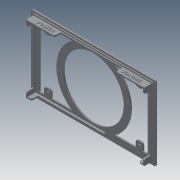
# Autodesk Inventor part: upper
Saved by Autodesk Inventor 2014 (Build 180170000, 170)
## iProperties
Created: 2014-09-06
Part Number: upper
Material: 一般
Document SubType Name: Modeling
Designer: Hideyuki Takei
Density: 1 g/cm^3
Appearance: 既定
Author: Hideyuki Takei
Autodesk Inventor part; units mm, degrees
ref_plane "YZ Plane" through (0, 0, 0) normal (1, 0, 0) x (0, 1, 0)
ref_plane "XZ Plane" through (0, 0, 0) normal (0, 1, 0) x (-1, 0, 0)
ref_plane "XY Plane" through (0, 0, 0) normal (0, 0, 1) x (1, 0, 0)
sketch "スケッチ2" plane through (0, 0, 0) normal (0, 1, 0) x (-1, 0, 0)
  line L0 (0, 0) -> (136, 0)
  line L1 (136, 0) -> (136, 81)
  line L2 (136, 81) -> (0, 81)
  line L3 (0, 81) -> (0, 0)
  dimension "d2" = 81
  dimension "d3" = 136
  constraints: 8 end point, 2 parallel, 1 horizontal, 1 perpendicular
  measures "d2" distance of L2.end L0.start
  measures "d3" distance of L1.end L2.end
extrude "押し出し1" add sketch "スケッチ2" along normal blind 1.5
sketch "スケッチ3" plane through (0, 0, 0) normal (0, 1, 0) x (-1, 0, 0)
  line L0 (5, 5) -> (131, 5)
  line L1 (131, 5) -> (131, 76)
  line L2 (131, 76) -> (5, 76)
  line L3 (5, 76) -> (5, 5)
  line L4 (136, 0) -> (136, 81) projected
  line L5 (136, 81) -> (0, 81) projected
  line L6 (132.5, 77.5) -> (126.5, 77.5)
  line L7 (126.5, 77.5) -> (126.5, 76)
  line L8 (126.5, 76) -> (132.5, 76)
  line L9 (132.5, 76) -> (132.5, 77.5)
  line L10 (131, 76) -> (132.5, 76)
  line L11 (132.5, 76) -> (132.5, 71)
  line L12 (132.5, 71) -> (131, 71)
  line L13 (131, 71) -> (131, 76)
  line L14 (131, 5) -> (132.5, 5)
  line L15 (132.5, 5) -> (132.5, 10)
  line L16 (132.5, 10) -> (131, 10)
  line L17 (131, 10) -> (131, 5)
  line L18 (132.5, 5) -> (126.5, 5)
  line L19 (126.5, 5) -> (126.5, 3.5)
  line L20 (126.5, 3.5) -> (132.5, 3.5)
  line L21 (132.5, 3.5) -> (132.5, 5)
  line L22 (5, 76) -> (3.5, 76)
  line L23 (3.5, 76) -> (3.5, 71)
  line L24 (3.5, 71) -> (5, 71)
  line L25 (5, 71) -> (5, 76)
  line L26 (3.5, 76) -> (9.5, 76)
  line L27 (9.5, 76) -> (9.5, 77.5)
  line L28 (9.5, 77.5) -> (3.5, 77.5)
  line L29 (3.5, 77.5) -> (3.5, 76)
  line L30 (5, 5) -> (3.5, 5)
  line L31 (3.5, 5) -> (3.5, 10)
  line L32 (3.5, 10) -> (5, 10)
  line L33 (5, 10) -> (5, 5)
  line L34 (3.5, 5) -> (9.5, 5)
  line L35 (9.5, 5) -> (9.5, 3.5)
  line L36 (9.5, 3.5) -> (3.5, 3.5)
  line L37 (3.5, 3.5) -> (3.5, 5)
  point P0 (0, 0)
  dimension "d6" = 126
  dimension "d7" = 71
  dimension "d8" = 5
  dimension "d9" = 5
  dimension "d10" = 1.5
  dimension "d11" = 1.5
  dimension "d12" = 5
  dimension "d13" = 6
  dimension "d14" = 0
  dimension "d17" = 1.5
  dimension "d18" = 1.5
  dimension "d19" = 6
  dimension "d20" = 5
  dimension "d21" = 5
  dimension "d22" = 1.5
  dimension "d23" = 1.5
  dimension "d24" = 6
  dimension "d25" = 6
  dimension "d26" = 1.5
  dimension "d27" = 1.5
  dimension "d28" = 5
  constraints: 72 end point, 18 parallel, 9 horizontal, 9 perpendicular, 1 point on line
  measures "d6" distance of L1.end L2.end
  measures "d7" distance of L0.end L1.end
  measures "d8" distance between parallel lines of L4 L1
  measures "d9" distance between parallel lines of L5 L2
  measures "d10" distance of L11.end L12.end
  measures "d11" distance of L8.end L6.start
  measures "d12" distance of L10.end L11.end
  measures "d13" distance of L6.start L6.end
  measures "d14" distance between parallel lines of L11 L9
  measures "d17" distance of L15.end L16.end
  measures "d18" distance of L20.end L14.end
  measures "d19" distance of L19.end L20.end
  measures "d20" distance of L14.end L15.end
  measures "d21" distance of L22.end L23.end
  measures "d22" distance of L23.end L24.end
  measures "d23" distance of L28.end L22.end
  measures "d24" distance of L27.end L28.end
  measures "d25" distance of L35.end L36.end
  measures "d26" distance of L34.end L35.end
  measures "d27" distance of L31.end L32.end
  measures "d28" distance of L30.end L31.end
extrude "押し出し2" add sketch "スケッチ3" against normal blind 9.01 contours L30 L31 L32 L3 | L0 L35 L36 L37 L30 | L0 L14 L21 L20 L19 | L24 L23 L22 L3 | L1 L16 L15 L14 | L22 L29 L28 L27 L2 | L1 L8 L11 L12 | L7 L6 L9 L8 L2
sketch "スケッチ5" plane through (0, 0, 0) normal (0, 1, 0) x (-1, 0, 0)
  line L0 (131, 76) -> (5, 76)
  line L1 (5, 76) -> (5, 5)
  line L2 (5, 5) -> (131, 5)
  line L3 (131, 5) -> (131, 76)
  line L4 (0, 81) -> (0, 0) projected
  line L5 (131, 76) -> (5, 76)
  line L6 (5, 76) -> (5, 77.5)
  line L7 (5, 77.5) -> (131, 77.5)
  line L8 (131, 77.5) -> (131, 76)
  line L9 (131, 5) -> (5, 5)
  line L10 (5, 5) -> (5, 3.5)
  line L11 (5, 3.5) -> (131, 3.5)
  line L12 (131, 3.5) -> (131, 5)
  line L13 (131, 77.5) -> (132.5, 77.5)
  line L14 (132.5, 77.5) -> (132.5, 3.5)
  line L15 (132.5, 3.5) -> (131, 3.5)
  line L16 (131, 3.5) -> (131, 77.5)
  line L17 (5, 77.5) -> (3.5, 77.5)
  line L18 (3.5, 77.5) -> (3.5, 3.5)
  line L19 (3.5, 3.5) -> (5, 3.5)
  line L20 (5, 3.5) -> (5, 77.5)
  dimension "d34" = 126
  dimension "d35" = 71
  dimension "d36" = 5
  dimension "d37" = 5
  dimension "d38" = 1.5
  dimension "d39" = 1.5
  dimension "d40" = 1.5
  dimension "d41" = 1.5
  dimension "d42" = 1.5
  dimension "d43" = 1.5
  constraints: 40 end point, 10 parallel, 5 horizontal, 5 perpendicular
  measures "d34" distance of L0.start L0.end
  measures "d35" distance of L2.end L0.start
  measures "d36" distance from line of L4.end L2
  measures "d37" distance between parallel lines of L4 L1
  measures "d38" distance of L5.end L6.end
  measures "d39" distance of L9.end L10.end
  measures "d40" distance of L14.end L15.end
  measures "d41" distance of L18.end L19.end
  measures "d42" distance between parallel lines of L19 L2
  measures "d43" distance between parallel lines of L18 L1
extrude "押し出し4" add sketch "スケッチ5" against normal blind 2 contours L8 L13 L14 L15 L12 L3 | L0 L6 L7 L8 | L1 L10 L19 L18 L17 L6 | L12 L11 L10 L2
sketch "スケッチ6" plane through (0, -2, 0) normal (0, -1, 0) x (1, 0, 0)
  line L0 (-126.5, 76) -> (-126.5, 77.5) projected
  line L1 (-126.5, 76) -> (-9.5, 76) projected
  line L2 (-9.5, 77.5) -> (-126.5, 77.5) projected
  line L3 (-126.5, 77.5) -> (-101.5, 77.5)
  line L4 (-101.5, 77.5) -> (-101.5, 76)
  line L5 (-101.5, 76) -> (-126.5, 76)
  line L6 (-126.5, 76) -> (-126.5, 77.5)
  line L7 (-9.5, 76) -> (-34.5, 76)
  line L8 (-34.5, 76) -> (-34.5, 77.5)
  line L9 (-34.5, 77.5) -> (-9.5, 77.5)
  line L10 (-9.5, 77.5) -> (-9.5, 76)
  point P0 (0, 0)
  dimension "d46" = 25
  dimension "d47" = 25
  constraints: 16 end point, 4 parallel, 2 horizontal, 2 perpendicular, 2 point on line
  measures "d46" distance of L0.end L3.end
  measures "d47" distance of L8.end L9.end
extrude "押し出し5" add sketch "スケッチ6" along normal blind 7 contours L0 L2 L4 L1 | L8 L2 L10 L1
sketch "スケッチ7" plane through (0, 0, 0) normal (0, 1, 0) x (-1, 0, 0)
  line L0 (9, 73.5) -> (127, 73.5)
  line L1 (127, 73.5) -> (127, 7.5)
  line L2 (127, 7.5) -> (9, 7.5)
  line L3 (9, 7.5) -> (9, 73.5)
  line L4 (136, 0) -> (136, 81) projected
  line L5 (136, 81) -> (0, 81) projected
  point P0 (0, 0)
  dimension "d50" = 66
  dimension "d51" = 118
  dimension "d52" = 9
  dimension "d53" = 7.5
  constraints: 8 end point, 2 parallel, 1 horizontal, 1 perpendicular
  measures "d50" distance of L0.end L1.end
  measures "d51" distance of L1.end L2.end
  measures "d52" distance between parallel lines of L1 L4
  measures "d53" distance between parallel lines of L5 L0
extrude "押し出し6" cut sketch "スケッチ7" along normal up to next
sketch "スケッチ8" plane through (0, 0, 0) normal (0, 1, 0) x (-1, 0, 0)
  circle A0 centre (68, 40.5) radius 33
  circle A1 centre (68, 40.5) radius 40.5
  line L0 (0, 81) -> (0, 0) projected
  line L1 (0, 0) -> (136, 0) projected
  dimension "d56" = 66
  dimension "d57" = 81
  dimension "d58" = 68
  dimension "d59" = 40.5
  constraints: 2 centre point, 1 coincident
  measures "d56" diameter of A0
  measures "d57" diameter of A1
  measures "d58" distance from line of L0 A0.centre
  measures "d59" distance from line of L1 A0.centre
extrude "押し出し7" add sketch "スケッチ8" along normal blind 1.5
sketch "スケッチ9" plane through (-132.5, 0, 77.5) normal (0, 0, 1) x (1, 0, 0)
  line L0 (129, 0) -> (129, -9.01) projected
  line L1 (0, 0) -> (129, 0) projected
  line L2 (0, 0) -> (129, 0)
  line L3 (129, 0) -> (129, -1)
  line L4 (129, -1) -> (0, -1)
  line L5 (0, -1) -> (0, 0)
  point P0 (132.5, 0)
  dimension "d62" = 1
  constraints: 8 end point, 2 parallel, 1 horizontal, 1 perpendicular, 1 point on line
  measures "d62" distance of L4.end L1.start
extrude "押し出し8" add sketch "スケッチ9" along normal blind 1.5
sketch "スケッチ10" plane through (-3.5, 0, 3.5) normal (0, 0, -1) x (-1, 0, 0)
  line L0 (129, 0) -> (129, -9.01) projected
  line L1 (0, 0) -> (129, 0)
  line L2 (129, 0) -> (129, -1)
  line L3 (129, -1) -> (0, -1)
  line L4 (0, -1) -> (0, 0)
  point P0 (-3.5, 0)
  dimension "d65" = 1
  constraints: 8 end point, 2 parallel, 1 horizontal, 1 perpendicular, 1 point on line
  measures "d65" distance of L1.end L2.end
extrude "押し出し9" add sketch "スケッチ10" along normal blind 1.5
sketch "スケッチ11" plane through (-3.5, -9.01, 10) normal (1, 0, 0) x (0, 0, -1)
  line L0 (-69, 9.01) -> (8, 9.01)
  line L1 (8, 9.01) -> (8, 8.01)
  line L2 (8, 8.01) -> (-69, 8.01)
  line L3 (-69, 8.01) -> (-69, 9.01)
  point P0 (10, 9.01)
  constraints: 8 end point, 2 parallel, 1 horizontal, 1 perpendicular
extrude "押し出し10" add sketch "スケッチ11" along normal blind 1.5
sketch "スケッチ12" plane through (-132.5, -9.01, 3.5) normal (-1, 0, 0) x (0, 0, 1)
  line L0 (-1.5, 9.01) -> (75.5, 9.01)
  line L1 (75.5, 9.01) -> (75.5, 8.01)
  line L2 (75.5, 8.01) -> (-1.5, 8.01)
  line L3 (-1.5, 8.01) -> (-1.5, 9.01)
  point P0 (-3.5, 9.01)
  constraints: 8 end point, 2 parallel, 1 horizontal, 1 perpendicular
extrude "押し出し11" add sketch "スケッチ12" along normal blind 1.5
sketch "スケッチ13" plane through (0, 1.5, 0) normal (0, 1, 0) x (1, 0, 0)
  line L0 (-44.5213, -7.5) -> (-9, -7.5) projected
  line L1 (-9, -7.5) -> (-9, -73.5) projected
  line L2 (-9, -73.5) -> (-44.5213, -73.5) projected
  line L3 (-91.4787, -73.5) -> (-127, -73.5) projected
  line L4 (-127, -73.5) -> (-127, -7.5) projected
  line L5 (-127, -7.5) -> (-91.4787, -7.5) projected
  line L6 (-122, -7.5) -> (-114, -7.5)
  line L7 (-114, -7.5) -> (-114, -15.5)
  line L8 (-114, -15.5) -> (-122, -15.5)
  line L9 (-122, -15.5) -> (-122, -7.5)
  line L10 (-122, -73.5) -> (-114, -73.5)
  line L11 (-114, -73.5) -> (-114, -65.5)
  line L12 (-114, -65.5) -> (-122, -65.5)
  line L13 (-122, -65.5) -> (-122, -73.5)
  line L14 (-14, -7.5) -> (-22, -7.5)
  line L15 (-22, -7.5) -> (-22, -15.5)
  line L16 (-22, -15.5) -> (-14, -15.5)
  line L17 (-14, -15.5) -> (-14, -7.5)
  line L18 (-14, -73.5) -> (-22, -73.5)
  line L19 (-22, -73.5) -> (-22, -65.5)
  line L20 (-22, -65.5) -> (-14, -65.5)
  line L21 (-14, -65.5) -> (-14, -73.5)
  circle A0 centre (-118, -12.5) radius 1.25
  circle A1 centre (-118, -68.5) radius 1.25
  circle A2 centre (-18, -12.5) radius 1.25
  circle A3 centre (-18, -68.5) radius 1.25
  dimension "d72" = 8
  dimension "d73" = 8
  dimension "d74" = 8
  dimension "d75" = 8
  dimension "d76" = 8
  dimension "d77" = 8
  dimension "d78" = 8
  dimension "d79" = 8
  dimension "d80" = 5
  dimension "d81" = 5
  dimension "d82" = 5
  dimension "d83" = 5
  dimension "d84" = 2.5
  dimension "d85" = 2.5
  dimension "d86" = 2.5
  dimension "d87" = 2.5
  dimension "d88" = 4
  dimension "d89" = 3
  dimension "d90" = 3
  dimension "d91" = 4
  dimension "d92" = 4
  dimension "d93" = 5
  dimension "d94" = 4
  dimension "d95" = 5
  constraints: 32 end point, 8 parallel, 4 centre point, 4 horizontal, 4 perpendicular, 4 point on line
  measures "d72" distance of L8.end L6.start
  measures "d73" distance of L12.end L10.start
  measures "d74" distance of L20.end L18.start
  measures "d75" distance of L16.end L14.start
  measures "d76" distance of L7.end L8.end
  measures "d77" distance of L11.end L12.end
  measures "d78" distance of L19.end L20.end
  measures "d79" distance of L15.end L16.end
  measures "d80" distance between parallel lines of L9 L4
  measures "d81" distance between parallel lines of L4 L13
  measures "d82" distance between parallel lines of L1 L17
  measures "d83" distance between parallel lines of L1 L21
  measures "d84" diameter of A3
  measures "d85" diameter of A1
  measures "d86" diameter of A0
  measures "d87" diameter of A2
  measures "d88" distance from line of L9 A0.centre
  measures "d89" distance from line of L8 A0.centre
  measures "d90" distance from line of L16 A2.centre
  measures "d91" distance from line of L15 A2.centre
  measures "d92" distance from line of L19 A3.centre
  measures "d93" distance from line of L2 A3.centre
  measures "d94" distance from line of L13 A1.centre
  measures "d95" distance from line of L3 A1.centre
extrude "押し出し12" add sketch "スケッチ13" against normal blind 1.5
fillet "フィレット1" radius 3 8 edges at (-14, 0.75, 65.5) (-22, 0.75, 65.5) (-114, 0.75, 65.5) (-122, 0.75, 65.5) (-114, 0.75, 15.5) (-122, 0.75, 15.5) (-14, 0.75, 15.5) (-22, 0.75, 15.5)
fillet "フィレット2" radius 1.5 8 edges at (0, 0.75, 81) (0, 0.75, 0) (-136, 0.75, 0) (-136, 0.75, 81) (-134, -0.5, 79) (-134, -0.5, 2) (-2, -0.5, 2) (-2, -0.5, 79)
sketch "スケッチ14" plane through (-9.5, -9.01, 77.5) normal (0, 0, 1) x (1, 0, 0)
  line L0 (6, 8.01) -> (-123, 8.01) projected
  line L1 (-123, 8.01) -> (-123, 0) projected
  line L2 (-114, 5.51) -> (-95.7285, 5.51) construction
  line L3 (-95.7285, 5.51) -> (-95.7285, 1.8625) construction
  line L4 (-95.7285, 1.8625) -> (-114, 1.8625) construction
  line L5 (-114, 1.8625) -> (-114, 5.51) construction
  line L6 (6, 8.01) -> (6, 0) projected
  line L7 (-22, 5.51) -> (-1.4737, 5.51) construction
  line L8 (-1.4737, 5.51) -> (-1.4737, 32.8525) construction
  line L9 (-1.4737, 32.8525) -> (-22, 32.8525) construction
  line L10 (-22, 32.8525) -> (-22, 5.51) construction
  spline S0 degree 2 poles (-110.9453, 4.3329) (-110.9453, 4.089) (-111.1013, 3.6465) (-111.2459, 3.4991) knots 0 0 0 1 2 2 2
  spline S1 degree 2 poles (-111.2459, 3.4991) (-111.3339, 3.4055) (-111.5494, 3.2523) (-111.6771, 3.1984) knots 0 0 0 1 2 2 2
  spline S2 degree 2 poles (-111.6771, 3.1984) (-111.8075, 3.1445) (-112.111, 3.0821) (-112.2982, 3.0821) knots 0 0 0 1 2 2 2
  line L11 (-112.2982, 3.0821) -> (-112.7577, 3.0821)
  line L12 (-112.7577, 3.0821) -> (-112.7577, 1.9363)
  line L13 (-112.7577, 1.9363) -> (-113.637, 1.9363)
  line L14 (-113.637, 1.9363) -> (-113.637, 5.4363)
  line L15 (-113.637, 5.4363) -> (-112.2784, 5.4363)
  spline S3 degree 2 poles (-112.2784, 5.4363) (-111.9777, 5.4363) (-111.5381, 5.3256) (-111.3594, 5.2065) knots 0 0 0 1 2 2 2
  spline S4 degree 2 poles (-111.3594, 5.2065) (-111.1609, 5.0732) (-110.9453, 4.6364) (-110.9453, 4.3329) knots 0 0 0 1 2 2 2
  spline S5 degree 2 poles (-111.8472, 4.3102) (-111.8472, 4.4606) (-111.9891, 4.6733) (-112.0855, 4.713) knots 0 0 0 1 2 2 2
  spline S6 degree 2 poles (-112.0855, 4.713) (-112.2103, 4.7669) (-112.4372, 4.7839) (-112.6329, 4.7839) knots 0 0 0 1 2 2 2
  line L16 (-112.6329, 4.7839) -> (-112.7577, 4.7839)
  line L17 (-112.7577, 4.7839) -> (-112.7577, 3.7345)
  line L18 (-112.7577, 3.7345) -> (-112.6953, 3.7345)
  spline S7 degree 2 poles (-112.6953, 3.7345) (-112.5733, 3.7345) (-112.3521, 3.7401) (-112.2699, 3.7543) knots 0 0 0 1 2 2 2
  spline S8 degree 2 poles (-112.2699, 3.7543) (-112.1989, 3.7657) (-112.0429, 3.8337) (-112.0004, 3.8763) knots 0 0 0 1 2 2 2
  spline S9 degree 2 poles (-112.0004, 3.8763) (-111.9096, 3.9614) (-111.8472, 4.1514) (-111.8472, 4.3102) knots 0 0 0 1 2 2 2
  spline S10 degree 2 poles (-107.2893, 3.6863) (-107.2893, 2.8354) (-108.1969, 1.8625) (-108.9854, 1.8625) knots 0 0 0 1 2 2 2
  spline S11 degree 2 poles (-108.9854, 1.8625) (-109.7767, 1.8625) (-110.6787, 2.8467) (-110.6787, 3.6863) knots 0 0 0 1 2 2 2
  spline S12 degree 2 poles (-110.6787, 3.6863) (-110.6787, 4.5286) (-109.7767, 5.51) (-108.9854, 5.51) knots 0 0 0 1 2 2 2
  spline S13 degree 2 poles (-108.9854, 5.51) (-108.1969, 5.51) (-107.2893, 4.5343) (-107.2893, 3.6863) knots 0 0 0 1 2 2 2
  spline S14 degree 2 poles (-108.1969, 3.6863) (-108.1969, 4.0011) (-108.3246, 4.4407) (-108.4352, 4.5797) knots 0 0 0 1 2 2 2
  spline S15 degree 2 poles (-108.4352, 4.5797) (-108.5458, 4.7243) (-108.8294, 4.8491) (-108.9826, 4.8491) knots 0 0 0 1 2 2 2
  spline S16 degree 2 poles (-108.9826, 4.8491) (-109.1442, 4.8491) (-109.408, 4.7329) (-109.53, 4.5854) knots 0 0 0 1 2 2 2
  spline S17 degree 2 poles (-109.53, 4.5854) (-109.6378, 4.4492) (-109.7711, 3.9982) (-109.7711, 3.6863) knots 0 0 0 1 2 2 2
  spline S18 degree 2 poles (-109.7711, 3.6863) (-109.7711, 3.3629) (-109.6434, 2.9375) (-109.5328, 2.7928) knots 0 0 0 1 2 2 2
  spline S19 degree 2 poles (-109.5328, 2.7928) (-109.4222, 2.6482) (-109.1357, 2.5234) (-108.9826, 2.5234) knots 0 0 0 1 2 2 2
  spline S20 degree 2 poles (-108.9826, 2.5234) (-108.8266, 2.5234) (-108.5373, 2.6567) (-108.4323, 2.7985) knots 0 0 0 1 2 2 2
  spline S21 degree 2 poles (-108.4323, 2.7985) (-108.3189, 2.9517) (-108.1969, 3.3572) (-108.1969, 3.6863) knots 0 0 0 1 2 2 2
  line L19 (-102.2549, 5.4363) -> (-103.1398, 1.9363)
  line L20 (-103.1398, 1.9363) -> (-104.1041, 1.9363)
  line L21 (-104.1041, 1.9363) -> (-104.6657, 4.1004)
  line L22 (-104.6657, 4.1004) -> (-105.2075, 1.9363)
  line L23 (-105.2075, 1.9363) -> (-106.1746, 1.9363)
  line L24 (-106.1746, 1.9363) -> (-107.0596, 5.4363)
  line L25 (-107.0596, 5.4363) -> (-106.1463, 5.4363)
  line L26 (-106.1463, 5.4363) -> (-105.6641, 3.0935)
  line L27 (-105.6641, 3.0935) -> (-105.0798, 5.4363)
  line L28 (-105.0798, 5.4363) -> (-104.2062, 5.4363)
  line L29 (-104.2062, 5.4363) -> (-103.6503, 3.0906)
  line L30 (-103.6503, 3.0906) -> (-103.1455, 5.4363)
  line L31 (-103.1455, 5.4363) -> (-102.2549, 5.4363)
  line L32 (-101.8209, 1.9363) -> (-101.8209, 5.4363)
  line L33 (-101.8209, 5.4363) -> (-99.4554, 5.4363)
  line L34 (-99.4554, 5.4363) -> (-99.4554, 4.7697)
  line L35 (-99.4554, 4.7697) -> (-100.9473, 4.7697)
  line L36 (-100.9473, 4.7697) -> (-100.9473, 4.1542)
  line L37 (-100.9473, 4.1542) -> (-99.5717, 4.1542)
  line L38 (-99.5717, 4.1542) -> (-99.5717, 3.4877)
  line L39 (-99.5717, 3.4877) -> (-100.9473, 3.4877)
  line L40 (-100.9473, 3.4877) -> (-100.9473, 2.6028)
  line L41 (-100.9473, 2.6028) -> (-99.4554, 2.6028)
  line L42 (-99.4554, 2.6028) -> (-99.4554, 1.9363)
  line L43 (-99.4554, 1.9363) -> (-101.8209, 1.9363)
  line L44 (-95.6264, 1.9363) -> (-96.6957, 1.9363)
  line L45 (-96.6957, 1.9363) -> (-97.6686, 3.2211)
  line L46 (-97.6686, 3.2211) -> (-97.9862, 3.2211)
  line L47 (-97.9862, 3.2211) -> (-97.9862, 1.9363)
  line L48 (-97.9862, 1.9363) -> (-98.8598, 1.9363)
  line L49 (-98.8598, 1.9363) -> (-98.8598, 5.4363)
  line L50 (-98.8598, 5.4363) -> (-97.453, 5.4363)
  spline S22 degree 2 poles (-97.453, 5.4363) (-97.1609, 5.4363) (-96.7297, 5.3625) (-96.5454, 5.2491) knots 0 0 0 1 2 2 2
  spline S23 degree 2 poles (-96.5454, 5.2491) (-96.3582, 5.1299) (-96.137, 4.7584) (-96.137, 4.4747) knots 0 0 0 1 2 2 2
  spline S24 degree 2 poles (-96.137, 4.4747) (-96.137, 4.0748) (-96.5, 3.5728) (-96.8035, 3.4253) knots 0 0 0 1 2 2 2
  line L51 (-96.8035, 3.4253) -> (-95.6264, 1.9363)
  spline S25 degree 2 poles (-97.0389, 4.3641) (-97.0389, 4.4974) (-97.141, 4.6875) (-97.2573, 4.7385) knots 0 0 0 1 2 2 2
  spline S26 degree 2 poles (-97.2573, 4.7385) (-97.3395, 4.7726) (-97.5409, 4.7924) (-97.6912, 4.7924) knots 0 0 0 1 2 2 2
  line L52 (-97.6912, 4.7924) -> (-97.9862, 4.7924)
  line L53 (-97.9862, 4.7924) -> (-97.9862, 3.8508)
  line L54 (-97.9862, 3.8508) -> (-97.7338, 3.8508)
  spline S27 degree 2 poles (-97.7338, 3.8508) (-97.5523, 3.8508) (-97.2942, 3.8961) (-97.2062, 3.9671) knots 0 0 0 1 2 2 2
  spline S28 degree 2 poles (-97.2062, 3.9671) (-97.1212, 4.0351) (-97.0389, 4.2166) (-97.0389, 4.3641) knots 0 0 0 1 2 2 2
  line L55 (-18.7156, 5.4363) -> (-19.9182, 1.9363)
  line L56 (-19.9182, 1.9363) -> (-20.8343, 1.9363)
  line L57 (-20.8343, 1.9363) -> (-22.0369, 5.4363)
  line L58 (-22.0369, 5.4363) -> (-21.1264, 5.4363)
  line L59 (-21.1264, 5.4363) -> (-20.3635, 3.0623)
  line L60 (-20.3635, 3.0623) -> (-19.6033, 5.4363)
  line L61 (-19.6033, 5.4363) -> (-18.7156, 5.4363)
  spline S29 degree 2 poles (-15.2042, 3.6863) (-15.2042, 2.8354) (-16.1118, 1.8625) (-16.9003, 1.8625) knots 0 0 0 1 2 2 2
  spline S30 degree 2 poles (-16.9003, 1.8625) (-17.6917, 1.8625) (-18.5936, 2.8467) (-18.5936, 3.6863) knots 0 0 0 1 2 2 2
  spline S31 degree 2 poles (-18.5936, 3.6863) (-18.5936, 4.5286) (-17.6917, 5.51) (-16.9003, 5.51) knots 0 0 0 1 2 2 2
  spline S32 degree 2 poles (-16.9003, 5.51) (-16.1118, 5.51) (-15.2042, 4.5343) (-15.2042, 3.6863) knots 0 0 0 1 2 2 2
  spline S33 degree 2 poles (-16.1118, 3.6863) (-16.1118, 4.0011) (-16.2395, 4.4407) (-16.3501, 4.5797) knots 0 0 0 1 2 2 2
  spline S34 degree 2 poles (-16.3501, 4.5797) (-16.4607, 4.7243) (-16.7443, 4.8491) (-16.8975, 4.8491) knots 0 0 0 1 2 2 2
  spline S35 degree 2 poles (-16.8975, 4.8491) (-17.0592, 4.8491) (-17.3229, 4.7329) (-17.4449, 4.5854) knots 0 0 0 1 2 2 2
  spline S36 degree 2 poles (-17.4449, 4.5854) (-17.5527, 4.4492) (-17.686, 3.9982) (-17.686, 3.6863) knots 0 0 0 1 2 2 2
  spline S37 degree 2 poles (-17.686, 3.6863) (-17.686, 3.3629) (-17.5583, 2.9375) (-17.4477, 2.7928) knots 0 0 0 1 2 2 2
  spline S38 degree 2 poles (-17.4477, 2.7928) (-17.3371, 2.6482) (-17.0506, 2.5234) (-16.8975, 2.5234) knots 0 0 0 1 2 2 2
  spline S39 degree 2 poles (-16.8975, 2.5234) (-16.7415, 2.5234) (-16.4522, 2.6567) (-16.3472, 2.7985) knots 0 0 0 1 2 2 2
  spline S40 degree 2 poles (-16.3472, 2.7985) (-16.2338, 2.9517) (-16.1118, 3.3572) (-16.1118, 3.6863) knots 0 0 0 1 2 2 2
  line L62 (-12.3481, 1.9363) -> (-14.6823, 1.9363)
  line L63 (-14.6823, 1.9363) -> (-14.6823, 5.4363)
  line L64 (-14.6823, 5.4363) -> (-13.8031, 5.4363)
  line L65 (-13.8031, 5.4363) -> (-13.8031, 2.6028)
  line L66 (-13.8031, 2.6028) -> (-12.3481, 2.6028)
  line L67 (-12.3481, 2.6028) -> (-12.3481, 1.9363)
  spline S41 degree 2 poles (-10.513, 1.8625) (-11.2192, 1.8625) (-11.9793, 2.5432) (-11.9793, 3.2012) knots 0 0 0 1 2 2 2
  line L68 (-11.9793, 3.2012) -> (-11.9793, 5.4363)
  line L69 (-11.9793, 5.4363) -> (-11.1001, 5.4363)
  line L70 (-11.1001, 5.4363) -> (-11.1001, 3.2523)
  spline S42 degree 2 poles (-11.1001, 3.2523) (-11.1001, 2.8864) (-10.825, 2.529) (-10.513, 2.529) knots 0 0 0 1 2 2 2
  spline S43 degree 2 poles (-10.513, 2.529) (-10.2095, 2.529) (-9.9259, 2.8722) (-9.9259, 3.2523) knots 0 0 0 1 2 2 2
  line L71 (-9.9259, 3.2523) -> (-9.9259, 5.4363)
  line L72 (-9.9259, 5.4363) -> (-9.0466, 5.4363)
  line L73 (-9.0466, 5.4363) -> (-9.0466, 3.2041)
  spline S44 degree 2 poles (-9.0466, 3.2041) (-9.0466, 2.5574) (-9.7869, 1.8625) (-10.513, 1.8625) knots 0 0 0 1 2 2 2
  line L74 (-4.7978, 1.9363) -> (-5.6714, 1.9363)
  line L75 (-5.6714, 1.9363) -> (-5.6714, 4.2564)
  line L76 (-5.6714, 4.2564) -> (-6.3067, 2.7588)
  line L77 (-6.3067, 2.7588) -> (-6.908, 2.7588)
  line L78 (-6.908, 2.7588) -> (-7.5434, 4.2564)
  line L79 (-7.5434, 4.2564) -> (-7.5434, 1.9363)
  line L80 (-7.5434, 1.9363) -> (-8.3716, 1.9363)
  line L81 (-8.3716, 1.9363) -> (-8.3716, 5.4363)
  line L82 (-8.3716, 5.4363) -> (-7.359, 5.4363)
  line L83 (-7.359, 5.4363) -> (-6.5818, 3.7089)
  line L84 (-6.5818, 3.7089) -> (-5.8104, 5.4363)
  line L85 (-5.8104, 5.4363) -> (-4.7978, 5.4363)
  line L86 (-4.7978, 5.4363) -> (-4.7978, 1.9363)
  line L87 (-4.0717, 1.9363) -> (-4.0717, 5.4363)
  line L88 (-4.0717, 5.4363) -> (-1.7062, 5.4363)
  line L89 (-1.7062, 5.4363) -> (-1.7062, 4.7697)
  line L90 (-1.7062, 4.7697) -> (-3.1981, 4.7697)
  line L91 (-3.1981, 4.7697) -> (-3.1981, 4.1542)
  line L92 (-3.1981, 4.1542) -> (-1.8225, 4.1542)
  line L93 (-1.8225, 4.1542) -> (-1.8225, 3.4877)
  line L94 (-1.8225, 3.4877) -> (-3.1981, 3.4877)
  line L95 (-3.1981, 3.4877) -> (-3.1981, 2.6028)
  line L96 (-3.1981, 2.6028) -> (-1.7062, 2.6028)
  line L97 (-1.7062, 2.6028) -> (-1.7062, 1.9363)
  line L98 (-1.7062, 1.9363) -> (-4.0717, 1.9363)
  point P0 (9.5, 9.01)
  dimension "d101" = 9
  dimension "d102" = 2.5
  dimension "d105" = 2.5
  dimension "d106" = 28
  constraints: 4 other
  measures "d101" distance from line of L1 L2.start
  measures "d102" distance from line of L0 L2.start
  measures "d105" distance from line of L0 L7.start
  measures "d106" distance from line of L6 L9.end
extrude "押し出し13" add sketch "スケッチ14" along normal blind 0.6
sketch "スケッチ15" plane through (0, -2, 0) normal (0, -1, 0) x (1, 0, 0)
  line L0 (-101.5, 77.5) -> (-101.5, 76) projected
  line L1 (-101.5, 76) -> (-34.5, 76) projected
  line L2 (-34.5, 77.5) -> (-101.5, 77.5) projected
  line L3 (-93, 77.5) -> (-43, 77.5)
  line L4 (-43, 77.5) -> (-43, 76)
  line L5 (-43, 76) -> (-93, 76)
  line L6 (-93, 76) -> (-93, 77.5)
  point P0 (0, 0)
  dimension "d107" = 50
  dimension "d108" = 8.5
  constraints: 8 end point, 2 parallel, 2 point on line, 1 horizontal, 1 perpendicular
  measures "d107" distance of L3.start L3.end
  measures "d108" distance from line of L0 L5.end
extrude "押し出し14" [suppressed]
fillet "フィレット3" radius 2 2 edges at (-101.5, -9, 76.75) (-34.5, -9, 76.75)
sketch "スケッチ16" plane through (0, -2, 0) normal (0, -1, 0) x (1, 0, 0)
  line L0 (-126.5, 3.5) -> (-9.5, 3.5) projected
  line L1 (-9.5, 5) -> (-54.5, 5)
  line L2 (-54.5, 5) -> (-54.5, 3.5)
  line L3 (-54.5, 3.5) -> (-9.5, 3.5)
  line L4 (-9.5, 3.5) -> (-9.5, 5)
  line L5 (-54.5, 3.5) -> (-9.5, 3.5)
  line L6 (-9.5, 3.5) -> (-9.5, 2)
  line L7 (-9.5, 2) -> (-54.5, 2)
  line L8 (-54.5, 2) -> (-54.5, 3.5)
  point P0 (0, 0)
  dimension "d111" = 45
  dimension "d114" = 1.5
  constraints: 16 end point, 4 parallel, 2 horizontal, 2 perpendicular, 1 point on line
  measures "d111" distance of L1.start L1.end
  measures "d114" distance of L7.end L2.end
extrude "押し出し15" cut sketch "スケッチ16" against normal blind 2
fillet "フィレット4" radius 2 6 edges at (-131.75, -9.01, 71) (-131.75, -9.01, 10) (-126.5, -9.01, 4.25) (-4.25, -9.01, 71) (-4.25, -9.01, 10) (-9.5, -9.01, 4.25)
equation "\"d52\" = 0.5 * d3 - 0.5 * d51"
equation "\"d53\" = 0.5 * d2 - 0.5 * d50"
equation "\"d58\" = 0.5 * d3"
equation "\"d59\" = 0.5 * d2"
